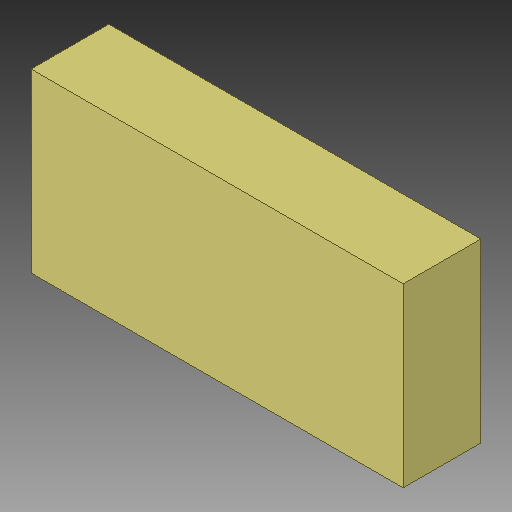
# Autodesk Inventor part: SILK_3V3_TAG
Saved by Autodesk Inventor 2018 (Build 220112000, 112)
## iProperties
Created: 2015-11-24
Part Number: SILK_3V3_TAG
Material: Generic
Document SubType Name: Modeling
Designer: PhillipD
Density: 1 g/cm^3
Appearance: SILK_3V3_TAG, SILK_3V3_TAG
Author: PhillipD
Autodesk Inventor part; units mm, degrees
ref_plane "YZ Plane" through (0, 0, 0) normal (1, 0, 0) x (0, 1, 0)
ref_plane "XZ Plane" through (0, 0, 0) normal (0, 1, 0) x (-1, 0, 0)
ref_plane "XY Plane" through (0, 0, 0) normal (0, 0, 1) x (1, 0, 0)
sketch "SILK_3V3_TAG, SILK_3V3_TAG_162" plane through (0, 0, 0) normal (0, 0, 1) x (1, 0, 0)
  line L0 (0, 2.2733) -> (4.7879, 2.2733)
  line L1 (4.7879, 2.2733) -> (4.7879, 0)
  line L2 (4.7879, 0) -> (0, 0)
  line L3 (0, 0) -> (0, 2.2733)
  constraints: 8 end point
extrude "Extrusion1" add sketch "SILK_3V3_TAG, SILK_3V3_TAG_162" along normal blind 1
body "Solid1"
